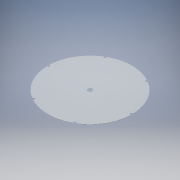
# Autodesk Inventor part: 2f2surf
Saved by Autodesk Inventor 2016 (Build 200138000, 138)
## iProperties
Company: HERA Project
Created: 2013-05-29
Part Number: 2f2surf
Material: Glass
Document SubType Name: Modeling
Designer: David DeBoer
Density: 2.18 g/cm^3
Description: Feed backplane conducting surface
Mass: 8147.17 g
Surface Area: 29543.6 cm^2
Volume: 3737.23 cm^3
Appearance: Clear
Author: David DeBoer
Title: Feed backplane surface
Autodesk Inventor part; units mm, degrees
ref_plane "YZ Plane" through (0, 0, 0) normal (1, 0, 0) x (0, 1, 0)
ref_plane "XZ Plane" through (0, 0, 0) normal (0, 1, 0) x (-1, 0, 0)
ref_plane "XY Plane" through (0, 0, 0) normal (0, 0, 1) x (1, 0, 0)
sketch "Sketch1" plane through (0, 0, 0) normal (0, 1, 0) x (-1, 0, 0)
  circle A0 centre (0.6883, 0.5378) radius 860
  point P0 (0, 0)
  dimension "d0" = 1720
  constraints: 1 centre point
  measures "d0" diameter of A0
extrude "Extrusion1" add sketch "Sketch1" along normal blind 2.54
sketch "Sketch2" plane through (-0.6883, 2.54, 0.5378) normal (0, 1, 0) x (1, 0, 0)
  circle A0 centre (0.6883, 0.5378) radius 45
  dimension "d7" = 90
  constraints: 1 centre point, 1 coincident
  measures "d7" diameter of A0
extrude "Extrusion2" cut sketch "Sketch2" against normal blind 25.4
sketch "Sketch3" plane through (-0.6883, 2.54, 0.5378) normal (0, 1, 0) x (1, 0, 0)
  circle A0 centre (0, 0) radius 860 projected
  line L0 (-893.9159, 16.958) -> (-826.0841, 16.958)
  line L1 (-826.0841, 16.958) -> (-826.0841, -16.958)
  line L2 (-826.0841, -16.958) -> (-893.9159, -16.958)
  line L3 (-893.9159, -16.958) -> (-893.9159, 16.958)
  line L4 (-860, 16.958) -> (-860, -16.958) construction
  line L5 (0, 0) -> (-860, 0) construction
  constraints: 12 end point, 3 midpoint, 2 parallel, 2 perpendicular, 1 horizontal, 1 horizontal alignment, 1 other
extrude "Extrusion3" cut sketch "Sketch3" against normal blind 10 contours L0 L1 L2 A0 | A0 L2 L3 L0 picked at (-837.3832, 1.8843)
pattern_circular "Circular Pattern1" count 6 over 360 about axis through (0, 2.54, 0) along (0, -1, 0) of "Extrusion3"
body "Solid1"
